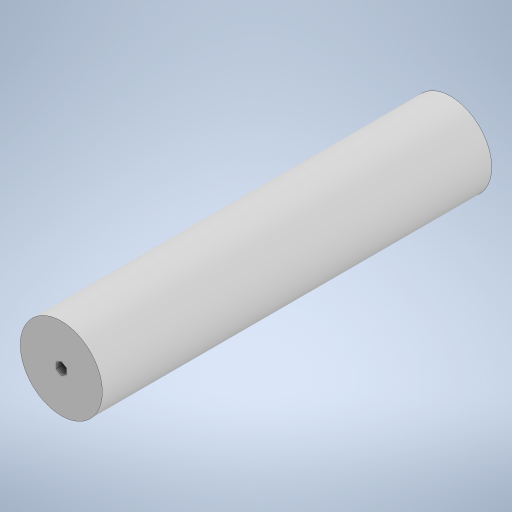
# Autodesk Inventor part: 4-bar intake roller
Saved by Autodesk Inventor 2023 (Build 270158030, 158C)
## iProperties
Created: 2022-07-18
Part Number: 4-bar intake roller
Material: Generic
Document SubType Name: Modeling
Designer: kt1040502
Density: 1 g/cm^3
Appearance: Default
Author: kt1040502
Autodesk Inventor part; units mm, degrees
ref_plane "YZ Plane" through (0, 0, 0) normal (1, 0, 0) x (0, 1, 0)
ref_plane "XZ Plane" through (0, 0, 0) normal (0, 1, 0) x (-1, 0, 0)
ref_plane "XY Plane" through (0, 0, 0) normal (0, 0, 1) x (1, 0, 0)
sketch "Sketch1" plane through (0, 0, 0) normal (0, 0, 1) x (1, 0, 0)
  circle A0 centre (0, 0) radius 50.8
  circle A1 centre (0, 0) radius 6.35
  line L0 (6.35, -3.6662) -> (0, -7.3323)
  line L1 (0, -7.3323) -> (-6.35, -3.6662)
  line L2 (-6.35, -3.6662) -> (-6.35, 3.6662)
  line L3 (-6.35, 3.6662) -> (0, 7.3323)
  line L4 (0, 7.3323) -> (6.35, 3.6662)
  line L5 (6.35, 3.6662) -> (6.35, -3.6662)
  point P0 (6.35, 0)
  dimension "d4" = 12.7
  dimension "d0" = 101.6
  constraints: 12 end point, 3 coincident, 1 centre point, 1 horizontal alignment, 1 midpoint, 15 other
  measures "d0" diameter of A0
extrude "Extrusion1" add sketch "Sketch1" along normal blind 482.6
body "Solid1"
